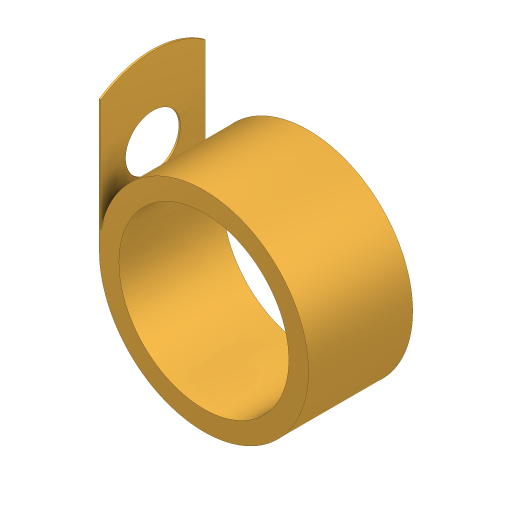
# Autodesk Inventor part: LCF  040 04 025S (on 10.35mm hub)
Saved by Autodesk Inventor 2023 (Build 270158000, 158)
## iProperties
Created: 2022-10-01
Part Number: LCF  040 04 025S (on 10.35mm hub)
Material: Generic
Document SubType Name: Modeling
Designer: david
Density: 1 g/cm^3
Appearance: Brass - Satin
Author: david
Autodesk Inventor part; units mm, degrees
ref_plane "YZ Plane" through (0, 0, 0) normal (1, 0, 0) x (0, 1, 0)
ref_plane "XZ Plane" through (0, 0, 0) normal (0, 1, 0) x (-1, 0, 0)
ref_plane "XY Plane" through (0, 0, 0) normal (0, 0, 1) x (1, 0, 0)
sketch "Sketch1" plane through (0, 0, 0) normal (0, 0, 1) x (1, 0, 0)
  circle A0 centre (0, 0) radius 5.175
  circle A1 centre (0, 0) radius 6.375
  line L0 (-6.375, 0) -> (-6.275, 0)
  line L1 (-6.275, 0) -> (-6.275, 9)
  line L2 (-6.275, 9) -> (-6.375, 9)
  line L3 (-6.375, 9) -> (-6.375, 0)
  point P0 (-6.275, 1.1247)
  dimension "d1" = 12.75
  dimension "d0" = 10.35
  dimension "d2" = 9
  dimension "d3" = 0.1
  constraints: 8 end point, 2 coincident, 2 parallel, 1 centre point, 1 horizontal, 1 perpendicular, 3 other
  measures "d0" diameter of A0
  measures "d2" distance of L2.end L0.start
  measures "d3" distance of L1.end L2.end
extrude "Extrusion1" add sketch "Sketch1" along normal blind 6.35
sketch "Sketch2" plane through (-6.375, 0, 0) normal (-1, 0, 0) x (0, 0, 1)
  line L0 (6.35, 1.1247) -> (6.35, 9) projected
  line L1 (0, 1.1247) -> (0, 9) projected
  arc A0 (6.35, 8.0079) -> (0, 7.9978) centre (3.1822, 3.4466) ccw
  circle A1 centre (3.175, 4.175) radius 1.675
  line L2 (0, 9) -> (6.35, 9) projected
  line L3 (0, 9) -> (6.35, 9)
  point P0 (0, 0)
  point P1 (3.1734, 9)
  point P2 (3.1894, 9)
  dimension "d6" = 4.825
  dimension "d7" = 3.35
  constraints: 3 point on circle, 2 centre point, 2 end point, 2 point on line, 1 horizontal
  measures "d6" distance of A1.centre point (3.173, 9)
  measures "d7" diameter of A1
extrude "Extrusion2" cut sketch "Sketch2" against normal up to surface (0.1 mm away)
body "Solid1"
